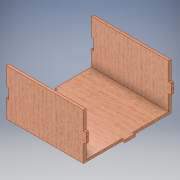
# Autodesk Inventor part: OpticalDeviceLensPart (1)
Saved by Autodesk Inventor 2017 (Build 210142000, 142)
## iProperties
Created: 2019-04-02
Part Number: OpticalDeviceLensPart (1)
Material: Generic
Document SubType Name: Modeling
Designer: Sharat
Density: 1 g/cm^3
Appearance: White Oak - Natural Medium Gloss
Author: Sharat
Autodesk Inventor part; units mm, degrees
ref_plane "YZ Plane" through (0, 0, 0) normal (1, 0, 0) x (0, 1, 0)
ref_plane "XZ Plane" through (0, 0, 0) normal (0, 1, 0) x (-1, 0, 0)
ref_plane "XY Plane" through (0, 0, 0) normal (0, 0, 1) x (1, 0, 0)
sketch "Sketch1" plane through (0, 0, 0) normal (0, 1, 0) x (-1, 0, 0)
  line L0 (0, 0) -> (-150, 0)
  line L1 (0, -170) -> (-150, -170)
  line L2 (-150, -170) -> (-150, -95)
  line L3 (-150, -95) -> (-155, -95)
  line L4 (-155, -95) -> (-155, -75)
  line L5 (-155, -75) -> (-150, -75)
  line L6 (-150, -75) -> (-150, 0)
  line L7 (0, -170) -> (0, -95)
  line L8 (0, -95) -> (-5, -95)
  line L9 (-5, -95) -> (-5, -75)
  line L10 (-5, -75) -> (0, -75)
  line L11 (0, -75) -> (0, 0)
  dimension "d0" = 150
  dimension "d1" = 170
  dimension "d2" = 5
  dimension "d3" = 5
  dimension "d4" = 75
  dimension "d5" = 75
  dimension "d6" = 20
  dimension "d9" = 0
  dimension "d10" = 75
  dimension "d11" = 5
  dimension "d12" = 75
  dimension "d13" = 20
  dimension "d14" = 150
  dimension "d15" = 0
  constraints: 24 end point, 8 perpendicular, 2 horizontal, 2 point on line, 2 vertical
  measures "d0" distance of L0.start L0.end
  measures "d1" distance of L1.start L0.start
  measures "d2" distance of L2.end L3.end
  measures "d3" distance of L4.end L5.end
  measures "d4" distance of L1.end L2.end
  measures "d5" distance of L5.end L0.end
  measures "d6" distance of L3.end L4.end
  measures "d9" distance from line of point (0, 0) L0
  measures "d10" distance of L1.start L7.end
  measures "d11" distance of L7.end L8.end
  measures "d12" distance of L10.end L0.start
  measures "d13" distance of L8.end L9.end
  measures "d14" distance between parallel lines of L6 L11
  measures "d15" distance from line of point (0, 0) L11
extrude "Extrusion1" add sketch "Sketch1" along normal blind 4.7625
sketch "Sketch2" plane through (0, 4.7625, 0) normal (0, 1, 0) x (1, 0, 0)
  line L0 (0, 0) -> (150, 0) projected
  line L1 (0, 0) -> (150, 0)
  line L2 (150, 0) -> (150, 4.7625)
  line L3 (150, 0) -> (150, 75) projected
  line L4 (150, 4.7625) -> (0, 4.7625)
  line L5 (0, 75) -> (0, 0) projected
  line L6 (0, 0) -> (0, 4.7625)
  line L7 (150, 170) -> (0, 170) projected
  line L8 (0, 170) -> (150, 170)
  line L9 (150, 170) -> (150, 165.2375)
  line L10 (150, 95) -> (150, 170) projected
  line L11 (150, 165.2375) -> (0, 165.2375)
  line L12 (0, 170) -> (0, 95) projected
  line L13 (0, 170) -> (0, 165.2375)
  dimension "d18" = 4.7625
  dimension "d19" = 4.7625
  constraints: 16 end point, 4 point on line, 3 perpendicular, 2 horizontal, 1 collinear
  measures "d18" distance of L0.end L2.end
  measures "d19" distance of L7.start L9.end
extrude "Extrusion2" add sketch "Sketch2" along normal blind 85.2375
sketch "Sketch3" plane through (0, 0, 0) normal (0, 0, 1) x (1, 0, 0)
  line L0 (0, 0) -> (0, 90) projected
  line L1 (0, 55) -> (5, 55)
  line L2 (5, 55) -> (5, 35)
  line L3 (5, 35) -> (0, 35)
  line L4 (0, 55) -> (0, 35)
  line L5 (0, 90) -> (150, 90) projected
  line L6 (0, 0) -> (150, 0) projected
  dimension "d22" = 20
  dimension "d23" = 5
  dimension "d24" = 35
  dimension "d25" = 35
  constraints: 8 end point, 2 perpendicular, 2 point on line, 1 collinear, 1 horizontal
  measures "d22" distance of L1.end L2.end
  measures "d23" distance of L1.start L1.end
  measures "d24" distance between parallel lines of L5 L1
  measures "d25" distance between parallel lines of L6 L3
extrude "Extrusion3" cut sketch "Sketch3" against normal blind 4.7625
sketch "Sketch4" plane through (150, 0, -170) normal (0, 0, -1) x (-1, 0, 0)
  line L0 (150, 0) -> (150, 90) projected
  line L1 (150, 35) -> (145, 35)
  line L2 (145, 35) -> (145, 55)
  line L3 (145, 55) -> (150, 55)
  line L4 (150, 55) -> (150, 35)
  line L5 (0, 90) -> (150, 90) projected
  line L6 (0, 0) -> (150, 0) projected
  dimension "d28" = 20
  dimension "d29" = 5
  dimension "d30" = 35
  dimension "d31" = 35
  constraints: 8 end point, 2 parallel, 1 horizontal, 1 perpendicular, 1 point on line
  measures "d28" distance of L1.end L2.end
  measures "d29" distance of L2.end L3.end
  measures "d30" distance between parallel lines of L5 L3
  measures "d31" distance between parallel lines of L6 L1
extrude "Extrusion4" cut sketch "Sketch4" against normal blind 4.7625
sketch "Sketch5" plane through (0, 0, 0) normal (0, 0, 1) x (1, 0, 0)
  line L0 (150, 0) -> (150, 90) projected
  line L1 (150, 55) -> (155, 55)
  line L2 (155, 55) -> (155, 35)
  line L3 (155, 35) -> (150, 35)
  line L4 (150, 35) -> (150, 55)
  line L5 (0, 0) -> (150, 0) projected
  line L6 (0, 90) -> (150, 90) projected
  dimension "d34" = 20
  dimension "d35" = 5
  dimension "d36" = 35
  dimension "d37" = 35
  constraints: 8 end point, 2 parallel, 1 horizontal, 1 perpendicular, 1 point on line
  measures "d34" distance of L1.end L2.end
  measures "d35" distance of L1.start L1.end
  measures "d36" distance between parallel lines of L5 L3
  measures "d37" distance between parallel lines of L6 L1
extrude "Extrusion5" add sketch "Sketch5" against normal blind 4.7625
sketch "Sketch6" plane through (150, 0, -170) normal (0, 0, -1) x (-1, 0, 0)
  line L0 (0, 55) -> (-5, 55) projected
  line L1 (0, 55) -> (-5, 55)
  line L2 (-5, 55) -> (-5, 35)
  line L3 (0, 4.7625) -> (0, 35) projected
  line L4 (-5, 35) -> (0, 35)
  line L5 (0, 35) -> (0, 55)
  point P0 (150, 0)
  constraints: 8 end point, 3 perpendicular, 1 horizontal
extrude "Extrusion6" add sketch "Sketch6" against normal blind 4.7625
fillet "Fillet1" radius 1 4 edges at (5, 35, -167.6188) (5, 55, -167.6188) (5, 55, -2.3813) (5, 35, -2.3813)
fillet "Fillet2" radius 1 4 edges at (155, 55, -2.3813) (155, 35, -2.3813) (155, 55, -167.6188) (155, 35, -167.6188)
hole "Hole1" at (155, 45.4891, -2.2612) direction (-1, 0, 0) diameter 2.5 depth 5 tip angle 118
hole "Hole2" at (155, 44.4165, -167.8579) direction (-1, 0, 0) diameter 2.5 depth 5 tip angle 118
body "Solid1"
